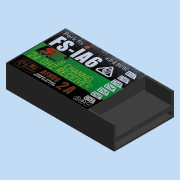
# Autodesk Inventor part: Flysky FS-iA6 Receiver
Saved by Autodesk Inventor 2022.3 (Build 263350030, 350C)
## iProperties
Created: 2022-09-05
Part Number: Flysky FS-iA6 Receiver
Material: Generic
Document SubType Name: Modeling
Designer: admin
Density: 1 g/cm^3
Appearance: Default
Author: admin
Autodesk Inventor part; units mm, degrees
ref_plane "YZ Plane" through (0, 0, 0) normal (1, 0, 0) x (0, 1, 0)
ref_plane "XZ Plane" through (0, 0, 0) normal (0, 1, 0) x (-1, 0, 0)
ref_plane "XY Plane" through (0, 0, 0) normal (0, 0, 1) x (1, 0, 0)
sketch "Sketch1" plane through (0, 0, 0) normal (0, 1, 0) x (-1, 0, 0)
  line L0 (26.6795, -25.7407) -> (-13.3205, -25.7407)
  line L1 (-13.3205, -25.7407) -> (-13.3205, -47.7407)
  line L2 (-13.3205, -47.7407) -> (26.6795, -47.7407)
  line L3 (26.6795, -47.7407) -> (26.6795, -25.7407)
  dimension "d0" = 40
  dimension "d1" = 22
  constraints: 8 end point, 2 parallel, 1 horizontal, 1 perpendicular
  measures "d0" distance of L2.end L1.end
  measures "d1" distance of L1.end L0.end
extrude "Extrusion1" add sketch "Sketch1" along normal blind 8.5
sketch "Sketch2" plane through (0, 8.5, 0) normal (0, 1, 0) x (1, 0, 0)
  line L0 (13.3205, 25.7407) -> (13.3205, 47.7407) projected
  line L1 (13.3205, 47.0907) -> (3.3205, 47.0907)
  line L2 (3.3205, 47.0907) -> (3.3205, 26.3907)
  line L3 (3.3205, 26.3907) -> (13.3205, 26.3907)
  line L4 (13.3205, 26.3907) -> (13.3205, 47.0907)
  line L5 (13.3205, 47.7407) -> (-26.6795, 47.7407) projected
  line L6 (-26.6795, 25.7407) -> (13.3205, 25.7407) projected
  point P0 (13.3205, 26.3907)
  point P1 (8.3205, 47.0907)
  dimension "d6" = 10
  dimension "d23" = 0.65
  dimension "d24" = 0.65
  constraints: 8 end point, 2 parallel, 1 horizontal, 1 midpoint, 1 perpendicular, 1 point on line
  measures "d6" distance between parallel lines of L0 L2
  measures "d23" distance between parallel lines of L6 L3
  measures "d24" distance from line of L5 point (8.321, 47.091)
extrude "Extrusion2" cut sketch "Sketch2" against normal blind 7.85
sketch "Sketch3" plane through (3.3205, 8.5, -26.3907) normal (1, 0, 0) x (0, 0, -1)
  line L0 (0.35, -4.25) -> (20.35, -4.25)
  line L1 (20.35, -4.25) -> (20.35, -5.85)
  line L2 (20.35, -5.85) -> (0.35, -5.85)
  line L3 (0.35, -5.85) -> (0.35, -4.25)
  line L4 (20.35, -5.05) -> (20.7, -5.05) construction
  line L5 (20.7, 0) -> (20.7, -7.85) construction
  line L6 (0.35, -5.05) -> (0, -5.05) construction
  line L7 (0, -7.85) -> (0, 0) construction
  line L8 (20.7, -7.85) -> (0, -7.85) construction
  dimension "d9" = 1.6
  dimension "d10" = 2
  dimension "d25" = 20
  constraints: 12 end point, 3 point on line, 2 horizontal, 2 midpoint, 2 parallel, 1 collinear, 1 perpendicular
  measures "d9" distance between parallel lines of L0 L2
  measures "d10" distance between parallel lines of L8 L2
  measures "d25" distance of L0.start L0.end
extrude "Extrusion3" add sketch "Sketch3" along normal up to surface (10 mm away)
sketch "Sketch4" plane through (3.3205, 4.25, -26.7407) normal (0, 1, 0) x (1, 0, 0)
  line L0 (0, 0) -> (10, 0) projected
  line L1 (10, 0) -> (10, 20) projected
  point P0 (-3.3205, -26.7407)
  point P1 (6.19, 2.5)
  dimension "d13" = 2.5
  dimension "d26" = 3.81
  measures "d13" distance from line of L0 point (6.19, 2.5)
  measures "d26" distance from line of L1 point (6.19, 2.5)
hole "Hole1" at (9.5105, 4.25, -29.2407) direction (0, -1, 0) diameter 1 depth 1.6
sketch "Sketch5" plane through (0, 8.5, 0) normal (0, 1, 0) x (1, 0, 0)
  line L0 (-26.3216, 47.7407) -> (3.3205, 47.7407) construction
  line L1 (3.3205, 47.7407) -> (3.3205, 25.7407) construction
  line L2 (3.3205, 25.7407) -> (-26.3216, 25.7407) construction
  line L3 (-26.3216, 25.7407) -> (-26.3216, 47.7407) construction
  line L4 (13.3205, 47.7407) -> (-26.6795, 47.7407) projected
  line L5 (3.3205, 26.3907) -> (3.3205, 47.0907) projected
  point P0 (3.3205, 36.7407)
  constraints: 2 midpoint, 1 point on line, 2 other
decal "Decal1"
body "Solid1"
